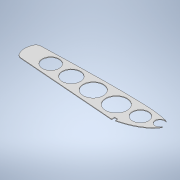
# Autodesk Inventor part: airfoil
Saved by Autodesk Inventor 2022 (Build 260153000, 153)
## iProperties
Created: 2021-03-06
Part Number: airfoil
Material: Generic
Document SubType Name: Modeling
Designer: Ferdinand Hubbard
Density: 1 g/cm^3
Appearance: Default
Author: Ferdinand Hubbard
Autodesk Inventor part; units mm, degrees
ref_plane "YZ Plane" through (0, 0, 0) normal (1, 0, 0) x (0, 1, 0)
ref_plane "XZ Plane" through (0, 0, 0) normal (0, 1, 0) x (-1, 0, 0)
ref_plane "XY Plane" through (0, 0, 0) normal (0, 0, 1) x (1, 0, 0)
sketch "Sketch1" plane through (0, 0, 0) normal (0, 1, 0) x (-1, 0, 0)
  line L0 (203.8757, 22.4313) -> (51.979, 34.2431)
  line L1 (362.8741, 0.9685) -> (367.8741, 0.9685)
  line L2 (367.8741, 0.9685) -> (367.8741, -4.0315)
  line L3 (367.8741, -4.0315) -> (362.8741, -4.0315)
  line L4 (362.8741, -4.0315) -> (362.8741, 0.9685)
  line L5 (211.4974, 21.8387) -> (210.0997, -8.5616) construction
  line L6 (46.4065, 34.5291) -> (51.4065, 34.5291)
  line L7 (51.4065, 34.5291) -> (51.4065, 29.5291)
  line L8 (51.4065, 29.5291) -> (46.4065, 29.5291)
  line L9 (46.4065, 29.5291) -> (46.4065, 34.5291)
  line L10 (46.4065, 34.5291) -> (51.4065, 29.5291) construction
  line L11 (51.4065, 34.5291) -> (46.4065, 29.5291) construction
  circle A0 centre (8.4978, 2.2571) radius 7.5
  circle A1 centre (139.6638, 8.2367) radius 14
  circle A2 centre (104.507, 9.4908) radius 15.5
  circle A3 centre (172.6846, 7.1168) radius 13
  circle A4 centre (259.3726, 4.4053) radius 7.5
  circle A5 centre (67.3244, 10.9193) radius 16.5
  line L12 (1.6385, 5.2903) -> (2.3233, 7.7402)
  line L13 (5.9301, -4.7897) -> (7.0011, -5.598)
  spline S0 degree 4 poles (51.979, 34.2431) (49.1051, 33.7566) (39.5332, 31.5872) (30.1137, 28.1904) (19.6059, 22.8943) (13.0923, 18.5073) (7.8605, 14.3051) (4.5473, 10.1712) (2.863, 8.0733) (2.0995, 6.7311) (1.9781, 6.5051) knots 0 0 0 0 0 0.341108 0.484452 0.62044 0.748582 0.868222 0.978476 1 1 1 1 1
  line L14 (5.0928, 12.3024) -> (-1.1366, 0.7079) construction
  arc A6 (5.0901, 10.4454) -> (0.4104, 1.7352) centre (14.6462, -0.301) ccw construction
  circle A7 centre (32.7718, 8.2367) radius 12.5
  circle A8 centre (281.2667, 3.3987) radius 6
  line L15 (227.2422, 19.7906) -> (370.1606, 1.1994)
  circle A9 centre (370.1606, 1.1994) radius 4 construction
  line L16 (367.8741, 0.9685) -> (366.8087, 1.6354)
  circle A10 centre (231.5291, 5.6854) radius 11.5
  circle A11 centre (231.5291, 5.6854) radius 4
  arc A12 (220.9876, 17.9175) -> (219.9803, -5.6004) centre (231.5291, 5.6854) ccw
  arc A13 (210.9733, -4.0867) -> (210.3341, 18.1827) centre (187.9502, 6.3964) ccw
  circle A14 centre (206.4716, 6.3964) radius 7.5
  spline S1 degree 4 poles (6.5182, -5.2336) (7.1415, -5.5888) (14.4853, -7.5093) (22.6172, -8.7121) (36.0297, -9.9499) (48.3532, -10.5062) (62.472, -10.893) (77.939, -11.061) (94.7612, -11.0653) (112.4597, -10.9248) (131.5397, -10.6367) (149.6391, -10.2913) (172.8653, -9.692) (180.7926, -9.5042) (198.4892, -8.9378) (204.2496, -8.7521) knots 0 0 0 0 0 0.110035 0.170402 0.235896 0.30593 0.379938 0.457319 0.537473 0.619837 0.703867 0.789037 0.873836 0.963807 0.963807 0.963807 0.963807 0.963807
  spline S2 degree 4 poles (225.8645, -8.0075) (229.0432, -7.891) (239.034, -7.5215) (249.3739, -7.0989) (267.437, -6.3281) (283.7249, -5.5266) (299.9849, -4.5949) (314.7321, -3.6133) (328.1645, -2.6483) (339.8259, -1.769) (350.0122, -1.0496) (357.5866, -0.5225) (364.806, -0.1794) (367.4848, -0.031) (370.1657, -0.0078) (369.9872, 0.0018) knots 0.038892 0.038892 0.038892 0.038892 0.038892 0.123258 0.214761 0.314941 0.412115 0.505682 0.594997 0.679292 0.757586 0.828586 0.890465 0.940044 1 1 1 1 1
  arc A15 (210.3341, 18.1827) -> (203.8757, 22.4313) centre (203.2555, 14.4554) ccw
  arc A16 (203.9596, -8.767) -> (210.9733, -4.0867) centre (203.6925, -0.7715) ccw
  arc A17 (227.2422, 19.7906) -> (220.9876, 17.9175) centre (226.2102, 11.8574) ccw
  arc A18 (219.9803, -5.6004) -> (225.9902, -8.0039) centre (225.7019, -0.0091) ccw
  line L17 (173.6294, -9.7393) -> (234.8699, -7.7649) construction
  arc A19 (179.7525, -9.5118) -> (228.7448, -7.9323) centre (-117.9879, 9986.0547) ccw construction
  line L18 (200.6438, -8.9311) -> (251.0851, -7.0838) construction
  arc A20 (205.6871, -8.7197) -> (246.0399, -7.2419) centre (-53.9768, 7633.4617) ccw construction
  point P0 (0, 0)
  point P1 (370, 0)
  point P2 (35.937, 30.0257)
  point P3 (27.0238, 26.4761)
  point P4 (19.2974, 22.4624)
  point P5 (12.8156, 18.139)
  point P6 (7.6237, 13.6489)
  point P7 (3.7499, 9.1521)
  point P8 (1.2115, 4.8535)
  point P9 (0.0668, 1.0195)
  point P10 (0.0003, -0.0638)
  point P11 (0.0755, -0.9849)
  point P12 (0.2106, -1.5356)
  point P13 (0.4302, -2.0122)
  point P14 (0.7739, -2.4345)
  point P15 (1.2488, -2.8423)
  point P16 (2.1566, -3.4383)
  point P17 (3.2773, -4.0196)
  point P18 (15.3669, -7.4261)
  point P19 (24.3167, -8.7706)
  point P20 (35.0526, -9.7678)
  point P21 (47.5438, -10.4262)
  point P22 (61.6814, -10.8267)
  point P23 (77.2847, -11.0213)
  point P24 (94.162, -11.0379)
  point P25 (112.1091, -10.9014)
  point P26 (130.911, -10.6315)
  point P27 (150.3435, -10.2474)
  point P28 (170.176, -9.7646)
  point P29 (190.1737, -9.1986)
  point P30 (267.1071, -6.3194)
  point P31 (284.4371, -5.4606)
  point P32 (300.619, -4.5258)
  point P33 (315.5184, -3.5432)
  point P34 (328.988, -2.5786)
  point P35 (340.8625, -1.7041)
  point P36 (350.9622, -0.9861)
  point P37 (359.0984, -0.4682)
  point P38 (365.0855, -0.1602)
  point P39 (368.7597, -0.0285)
  point P40 (369.9872, 0.0018)
  point P41 (48.9065, 32.0291)
  point P42 (112.1091, -11.9485)
  point P43 (1.9781, 6.5051)
  point P44 (51.4065, 34.1414)
  point P45 (46.4065, 33.0501)
  point P46 (224.3778, 20.1632)
  point P47 (207.7602, 22.1293)
  point P48 (204.2496, -8.7521)
  point P49 (225.8645, -8.0075)
  dimension "d8" = 160
  dimension "d26" = 5
  dimension "d27" = 5
  dimension "d36" = 5
  dimension "d37" = 5
  dimension "d50" = 368.7594
  dimension "d51" = 15
  dimension "d52" = 28
  dimension "d53" = 31
  dimension "d54" = 26
  dimension "d57" = 15
  dimension "d59" = 33
  dimension "d65" = 44.6693
  dimension "d66" = 25
  dimension "d67" = 12
  dimension "d68" = 160
  dimension "d69" = 8
  dimension "d70" = 23
  dimension "d71" = 8
  dimension "d73" = 15
  dimension "d74" = 8
  dimension "d75" = 8
  dimension "d76" = 8
  constraints: 38 end point, 21 centre point, 21 point on circle, 8 midpoint, 6 tangent, 5 point on line, 4 parallel, 3 coincident, 2 horizontal, 2 perpendicular, 1 equal radius, 45 other
  measures "d8" distance of L5.start L0.end
  measures "d26" distance of L2.end L3.end
  measures "d27" distance of L1.end L2.end
  measures "d36" distance of L7.end L8.end
  measures "d37" distance of L6.end L7.end
  measures "d50" distance of point (368.76, -0.028) point (0, -0.064)
  measures "d51" diameter of A0
  measures "d52" diameter of A1
  measures "d53" diameter of A2
  measures "d54" diameter of A3
  measures "d57" diameter of A4
  measures "d59" diameter of A5
  measures "d65" vertical distance of point (47.544, -10.426) L0.end
  measures "d66" diameter of A7
  measures "d67" diameter of A8
  measures "d68" distance of L5.start L15.end
  measures "d69" diameter of A9
  measures "d70" diameter of A10
  measures "d71" diameter of A11
  measures "d73" diameter of A14
  measures "d74" radius of A15
  measures "d75" radius of A16
  measures "d76" radius of A17
extrude "Extrusion4" add sketch "Sketch1" along normal blind 1 contours A15 A13 A14 A16 S1 L13 A0 L12 S0 L9 L8 L7 L0 | A13 A14 picked at (208.4876, 6.0855)
body "Solid4"
